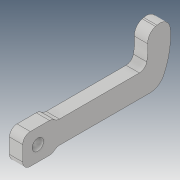
# Autodesk Inventor part: topArm
Saved by Autodesk Inventor 2018 (Build 220112000, 112)
## iProperties
Created: 2020-03-01
Part Number: topArm
Material: Generic
Document SubType Name: Modeling
Designer: anirudh
Density: 1 g/cm^3
Appearance: Default
Author: anirudh
Autodesk Inventor part; units mm, degrees
ref_plane "YZ Plane" through (0, 0, 0) normal (1, 0, 0) x (0, 1, 0)
ref_plane "XZ Plane" through (0, 0, 0) normal (0, 1, 0) x (-1, 0, 0)
ref_plane "XY Plane" through (0, 0, 0) normal (0, 0, 1) x (1, 0, 0)
sketch "Sketch1" plane through (0, 0, 0) normal (1, 0, 0) x (0, 1, 0)
  arc A0 (-32.8405, -38.3954) -> (-8.3696, -42.2273) centre (-16.2814, -12.7) ccw
  line L0 (-10.8348, -33.0268) -> (-8.3696, -42.2273)
  line L1 (-16.2814, -12.7) -> (18.6985, -12.7) construction
  line L2 (-16.2814, -12.7) -> (20.3214, -12.7) construction
  line L3 (-32.8405, 6.2103) -> (-32.8405, -38.3954)
  line L4 (-23.3155, 6.2103) -> (-23.3155, -32.5335)
  arc A1 (-23.3155, -32.5335) -> (-10.8348, -33.0268) centre (-16.2814, -12.7) ccw
  line L5 (-23.3155, 6.2103) -> (-23.3155, 0.4826)
  line L6 (-32.8405, 0.4826) -> (-32.8405, 6.2103)
  circle A2 centre (-28.078, 12.5603) radius 2.413
  line L7 (-34.428, 12.5603) -> (-34.428, 18.9103)
  line L8 (-34.428, 18.9103) -> (-28.078, 18.9103)
  line L9 (-34.428, 18.9103) -> (-21.728, 18.9103)
  line L10 (-21.728, 18.9103) -> (-21.728, 6.2103)
  line L11 (-34.428, 6.2103) -> (-34.428, 18.9103)
  line L12 (-21.728, 6.2103) -> (-23.3155, 6.2103)
  line L13 (-32.8405, 6.2103) -> (-34.428, 6.2103)
  point P0 (88.5698, 0)
  constraints: 28 end point, 4 parallel, 4 point on circle, 3 centre point, 3 horizontal, 2 vertical, 1 coincident, 1 perpendicular, 1 point on line
extrude "Extrusion3" add sketch "Sketch1" along normal blind 5.588
fillet "Fillet3" radius 4.445 2 edges at (2.794, -10.8348, -33.0268) (2.794, -8.3696, -42.2273)
fillet "Fillet4" radius 6.35 1 edges at (2.794, -32.8405, -38.3954)
fillet "Fillet5" radius 3.175 7 edges at (2.794, -23.3155, -32.5335) (2.794, -32.8405, 6.2103) (2.794, -34.428, 6.2103) (2.794, -23.3155, 6.2103) (2.794, -21.728, 6.2103) (2.794, -21.728, 18.9103) (2.794, -34.428, 18.9103)
body "Solid2"
